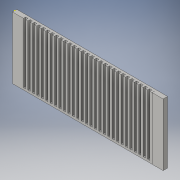
# Autodesk Inventor part: ModuleHolderReal
Saved by Autodesk Inventor 2016 (Build 200138000, 138)
## iProperties
Created: 2017-01-25
Part Number: ModuleHolderReal
Material: Generic
Document SubType Name: Modeling
Designer: RoboticsUser
Density: 1 g/cm^3
Appearance: Default
Author: RoboticsUser
Autodesk Inventor part; units mm, degrees
ref_plane "YZ Plane" through (0, 0, 0) normal (1, 0, 0) x (0, 1, 0)
ref_plane "XZ Plane" through (0, 0, 0) normal (0, 1, 0) x (-1, 0, 0)
ref_plane "XY Plane" through (0, 0, 0) normal (0, 0, 1) x (1, 0, 0)
sketch "Sketch1" plane through (0, 0, 0) normal (0, 0, 1) x (1, 0, 0)
  line L0 (0, 0) -> (215.9, 0)
  line L1 (215.9, 0) -> (215.9, -88.9)
  line L2 (215.9, -88.9) -> (0, -88.9)
  line L3 (0, -88.9) -> (0, 0)
  dimension "d0" = 215.9
  dimension "d1" = 88.9
  constraints: 8 end point, 2 parallel, 1 horizontal, 1 perpendicular
  measures "d0" distance of L1.end L2.end
  measures "d1" distance of L0.end L1.end
extrude "Extrusion1" add sketch "Sketch1" along normal blind 3.175
sketch "Sketch2" plane through (0, 0, 3.175) normal (0, 0, 1) x (1, 0, 0)
  line L0 (0, 0) -> (15.875, 0)
  line L1 (15.875, 0) -> (15.875, -88.9)
  line L2 (15.875, -88.9) -> (0, -88.9)
  line L3 (0, -88.9) -> (0, 0)
  dimension "d4" = 15.875
  dimension "d5" = 88.9
  constraints: 8 end point, 2 parallel, 1 horizontal, 1 perpendicular
  measures "d4" distance of L1.end L2.end
  measures "d5" distance of L0.end L1.end
extrude "Extrusion2" add sketch "Sketch2" along normal blind 3.175
sketch "Sketch3" plane through (0, 0, 3.175) normal (0, 0, 1) x (1, 0, 0)
  line L0 (215.9, -88.9) -> (0, -88.9) projected
  line L1 (15.8666, -88.9) -> (19.0416, -88.9)
  line L2 (19.0416, -88.9) -> (19.0416, -85.725)
  line L3 (19.0416, -85.725) -> (15.8666, -85.725)
  line L4 (15.8666, -85.725) -> (15.8666, -88.9)
  point P0 (0, 0)
  dimension "d8" = 3.175
  dimension "d9" = 3.175
  constraints: 8 end point, 2 parallel, 1 horizontal, 1 perpendicular, 1 point on line
  measures "d8" distance of L3.end L2.end
  measures "d9" distance of L2.end L1.end
extrude "Extrusion3" add sketch "Sketch3" along normal blind 3.175
sketch "Sketch4" plane through (0, 0, 3.175) normal (0, 0, 1) x (1, 0, 0)
  line L0 (19.0416, -85.725) -> (19.0416, -88.9) projected
  line L1 (19.0416, -88.9) -> (22.2166, -88.9)
  line L2 (22.2166, -88.9) -> (22.2166, 0)
  line L3 (22.2166, 0) -> (19.0416, 0)
  line L4 (19.0416, 0) -> (19.0416, -88.9)
  point P0 (0, 0)
  dimension "d12" = 3.175
  dimension "d13" = 88.9
  constraints: 8 end point, 2 parallel, 1 horizontal, 1 perpendicular
  measures "d12" distance of L3.end L2.end
  measures "d13" distance of L2.end L1.end
extrude "Extrusion4" add sketch "Sketch4" along normal blind 3.175
sketch "Sketch5" plane through (0, 0, 3.175) normal (0, 0, 1) x (1, 0, 0)
  line L0 (215.9, -88.9) -> (0, -88.9) projected
  line L1 (22.2165, -88.9) -> (25.3915, -88.9)
  line L2 (25.3915, -88.9) -> (25.3915, -85.725)
  line L3 (25.3915, -85.725) -> (22.2165, -85.725)
  line L4 (22.2165, -85.725) -> (22.2165, -88.9)
  point P0 (0, 0)
  dimension "d16" = 3.175
  dimension "d17" = 3.175
  constraints: 8 end point, 2 parallel, 1 horizontal, 1 perpendicular, 1 point on line
  measures "d16" distance of L3.end L2.end
  measures "d17" distance of L2.end L1.end
extrude "Extrusion5" add sketch "Sketch5" along normal blind 3.175
sketch "Sketch6" plane through (0, 0, 3.175) normal (0, 0, 1) x (1, 0, 0)
  point P0 (0, 0)
sketch "Sketch7" plane through (0, 0, 3.175) normal (0, 0, 1) x (1, 0, 0)
  line L0 (25.3915, -85.725) -> (25.3915, -88.9) projected
  line L1 (25.3915, -88.9) -> (28.5665, -88.9)
  line L2 (28.5665, -88.9) -> (28.5665, 0)
  line L3 (28.5665, 0) -> (25.3915, 0)
  line L4 (25.3915, 0) -> (25.3915, -88.9)
  point P0 (0, 0)
  dimension "d20" = 3.175
  dimension "d21" = 88.9
  constraints: 8 end point, 2 parallel, 1 horizontal, 1 perpendicular
  measures "d20" distance of L3.end L2.end
  measures "d21" distance of L2.end L1.end
extrude "Extrusion6" add sketch "Sketch7" along normal blind 3.175
sketch "Sketch8" plane through (0, 0, 3.175) normal (0, 0, 1) x (1, 0, 0)
  line L0 (28.5665, 0) -> (28.5665, -88.9) projected
  line L1 (28.5665, -88.9) -> (31.7415, -88.9)
  line L2 (31.7415, -88.9) -> (31.7415, -85.725)
  line L3 (31.7415, -85.725) -> (28.5665, -85.725)
  line L4 (28.5665, -85.725) -> (28.5665, -88.9)
  point P0 (0, 0)
  dimension "d24" = 3.175
  dimension "d25" = 3.175
  constraints: 8 end point, 2 parallel, 1 horizontal, 1 perpendicular
  measures "d24" distance of L3.end L2.end
  measures "d25" distance of L2.end L1.end
extrude "Extrusion7" add sketch "Sketch8" along normal blind 3.175
sketch "Sketch9" plane through (0, 0, 3.175) normal (0, 0, 1) x (1, 0, 0)
  line L0 (31.7415, -85.725) -> (31.7415, -88.9) projected
  line L1 (31.7415, -88.9) -> (34.9165, -88.9)
  line L2 (34.9165, -88.9) -> (34.9165, 0)
  line L3 (34.9165, 0) -> (31.7415, 0)
  line L4 (31.7415, 0) -> (31.7415, -88.9)
  point P0 (0, 0)
  dimension "d28" = 3.175
  dimension "d29" = 88.9
  constraints: 8 end point, 2 parallel, 1 horizontal, 1 perpendicular
  measures "d28" distance of L3.end L2.end
  measures "d29" distance of L2.end L1.end
extrude "Extrusion8" add sketch "Sketch9" along normal blind 3.175
sketch "Sketch10" plane through (0, 0, 3.175) normal (0, 0, 1) x (1, 0, 0)
  line L0 (215.9, -88.9) -> (215.9, 0) projected
  line L1 (215.9, -88.9) -> (200.025, -88.9)
  line L2 (200.025, -88.9) -> (200.025, 0)
  line L3 (200.025, 0) -> (215.9, 0)
  line L4 (215.9, 0) -> (215.9, -88.9)
  point P0 (0, 0)
  dimension "d32" = 15.875
  dimension "d33" = 88.9
  constraints: 8 end point, 2 parallel, 1 horizontal, 1 perpendicular
  measures "d32" distance of L2.end L3.end
  measures "d33" distance of L1.end L2.end
extrude "Extrusion9" add sketch "Sketch10" along normal blind 3.175
sketch "Sketch11" plane through (0, 0, 3.175) normal (0, 0, 1) x (1, 0, 0)
  line L0 (34.9165, 0) -> (34.9165, -88.9) projected
  line L1 (34.9165, -88.9) -> (38.0915, -88.9)
  line L2 (38.0915, -88.9) -> (38.0915, -85.725)
  line L3 (38.0915, -85.725) -> (34.9165, -85.725)
  line L4 (34.9165, -85.725) -> (34.9165, -88.9)
  point P0 (0, 0)
  dimension "d36" = 3.175
  dimension "d37" = 3.175
  constraints: 8 end point, 2 parallel, 1 horizontal, 1 perpendicular
  measures "d36" distance of L3.end L2.end
  measures "d37" distance of L2.end L1.end
extrude "Extrusion10" add sketch "Sketch11" along normal blind 3.175
sketch "Sketch12" plane through (0, 0, 3.175) normal (0, 0, 1) x (1, 0, 0)
  line L0 (38.0915, -88.9) -> (200.025, -88.9) projected
  line L1 (38.0915, -88.9) -> (41.2665, -88.9)
  line L2 (41.2665, -88.9) -> (41.2665, 0)
  line L3 (41.2665, 0) -> (38.0915, 0)
  line L4 (38.0915, 0) -> (38.0915, -88.9)
  point P0 (0, 0)
  dimension "d40" = 3.175
  dimension "d41" = 88.9
  constraints: 8 end point, 2 parallel, 1 horizontal, 1 perpendicular
  measures "d40" distance of L3.end L2.end
  measures "d41" distance of L2.end L1.end
extrude "Extrusion11" add sketch "Sketch12" along normal blind 3.175
sketch "Sketch13" plane through (0, 0, 3.175) normal (0, 0, 1) x (1, 0, 0)
  line L0 (41.2665, -88.9) -> (200.025, -88.9) projected
  line L1 (41.2665, -88.9) -> (44.4415, -88.9)
  line L2 (44.4415, -88.9) -> (44.4415, -85.725)
  line L3 (44.4415, -85.725) -> (41.2665, -85.725)
  line L4 (41.2665, -85.725) -> (41.2665, -88.9)
  point P0 (0, 0)
  dimension "d44" = 3.175
  dimension "d45" = 3.175
  constraints: 8 end point, 2 parallel, 1 horizontal, 1 perpendicular
  measures "d44" distance of L3.end L2.end
  measures "d45" distance of L2.end L1.end
extrude "Extrusion12" add sketch "Sketch13" along normal blind 3.175
sketch "Sketch14" plane through (0, 0, 3.175) normal (0, 0, 1) x (1, 0, 0)
  line L0 (44.4415, -88.9) -> (47.6165, -88.9)
  line L1 (47.6165, -88.9) -> (47.6165, 0)
  line L2 (47.6165, 0) -> (44.4415, 0)
  line L3 (44.4415, 0) -> (44.4415, -88.9)
  point P0 (0, 0)
  dimension "d48" = 3.175
  dimension "d49" = 88.9
  constraints: 8 end point, 2 parallel, 1 horizontal, 1 perpendicular
  measures "d48" distance of L2.end L1.end
  measures "d49" distance of L1.end L0.end
extrude "Extrusion13" add sketch "Sketch14" along normal blind 3.175
sketch "Sketch15" plane through (0, 0, 3.175) normal (0, 0, 1) x (1, 0, 0)
  line L0 (47.6165, -88.9) -> (200.025, -88.9) projected
  line L1 (47.6165, -88.9) -> (50.7915, -88.9)
  line L2 (50.7915, -88.9) -> (50.7915, -85.725)
  line L3 (50.7915, -85.725) -> (47.6165, -85.725)
  line L4 (47.6165, -85.725) -> (47.6165, -88.9)
  point P0 (0, 0)
  dimension "d52" = 3.175
  dimension "d53" = 3.175
  constraints: 8 end point, 2 parallel, 1 horizontal, 1 perpendicular
  measures "d52" distance of L3.end L2.end
  measures "d53" distance of L2.end L1.end
extrude "Extrusion14" add sketch "Sketch15" along normal blind 3.175
sketch "Sketch16" plane through (0, 0, 3.175) normal (0, 0, 1) x (1, 0, 0)
  line L0 (50.7915, -88.9) -> (200.025, -88.9) projected
  line L1 (50.7915, -88.9) -> (53.9665, -88.9)
  line L2 (53.9665, -88.9) -> (53.9665, 0)
  line L3 (53.9665, 0) -> (50.7915, 0)
  line L4 (50.7915, 0) -> (50.7915, -88.9)
  point P0 (0, 0)
  dimension "d56" = 3.175
  dimension "d57" = 88.9
  constraints: 8 end point, 2 parallel, 1 horizontal, 1 perpendicular
  measures "d56" distance of L3.end L2.end
  measures "d57" distance of L2.end L1.end
extrude "Extrusion15" add sketch "Sketch16" along normal blind 3.175
sketch "Sketch17" plane through (0, 0, 3.175) normal (0, 0, 1) x (1, 0, 0)
  line L0 (53.9665, -88.9) -> (200.025, -88.9) projected
  line L1 (53.9665, -88.9) -> (57.1415, -88.9)
  line L2 (57.1415, -88.9) -> (57.1415, -85.725)
  line L3 (57.1415, -85.725) -> (53.9665, -85.725)
  line L4 (53.9665, -85.725) -> (53.9665, -88.9)
  point P0 (0, 0)
  dimension "d60" = 3.175
  dimension "d61" = 3.175
  constraints: 8 end point, 2 parallel, 1 horizontal, 1 perpendicular
  measures "d60" distance of L3.end L2.end
  measures "d61" distance of L2.end L1.end
extrude "Extrusion16" add sketch "Sketch17" along normal blind 3.175
sketch "Sketch18" plane through (0, 0, 3.175) normal (0, 0, 1) x (1, 0, 0)
  line L0 (57.1415, -85.725) -> (57.1415, -88.9) projected
  line L1 (57.1415, -88.9) -> (60.3165, -88.9)
  line L2 (60.3165, -88.9) -> (60.3165, 0)
  line L3 (60.3165, 0) -> (57.1415, 0)
  line L4 (57.1415, 0) -> (57.1415, -88.9)
  point P0 (0, 0)
  dimension "d64" = 3.175
  dimension "d65" = 88.9
  constraints: 8 end point, 2 parallel, 1 horizontal, 1 perpendicular
  measures "d64" distance of L3.end L2.end
  measures "d65" distance of L2.end L1.end
extrude "Extrusion17" add sketch "Sketch18" along normal blind 3.175
sketch "Sketch19" plane through (0, 0, 3.175) normal (0, 0, 1) x (1, 0, 0)
  line L0 (60.3165, -88.9) -> (200.025, -88.9) projected
  line L1 (60.3165, -88.9) -> (63.4915, -88.9)
  line L2 (63.4915, -88.9) -> (63.4915, -85.725)
  line L3 (63.4915, -85.725) -> (60.3165, -85.725)
  line L4 (60.3165, -85.725) -> (60.3165, -88.9)
  point P0 (0, 0)
  dimension "d68" = 3.175
  dimension "d69" = 3.175
  constraints: 8 end point, 2 parallel, 1 horizontal, 1 perpendicular
  measures "d68" distance of L3.end L2.end
  measures "d69" distance of L2.end L1.end
extrude "Extrusion18" add sketch "Sketch19" along normal blind 3.175
sketch "Sketch20" plane through (0, 0, 3.175) normal (0, 0, 1) x (1, 0, 0)
  line L0 (63.4915, -85.725) -> (63.4915, -88.9) projected
  line L1 (63.4915, -88.9) -> (66.6665, -88.9)
  line L2 (66.6665, -88.9) -> (66.6665, 0)
  line L3 (66.6665, 0) -> (63.4915, 0)
  line L4 (63.4915, 0) -> (63.4915, -88.9)
  point P0 (0, 0)
  dimension "d72" = 3.175
  dimension "d73" = 88.9
  constraints: 8 end point, 2 parallel, 1 horizontal, 1 perpendicular
  measures "d72" distance of L3.end L2.end
  measures "d73" distance of L2.end L1.end
extrude "Extrusion19" add sketch "Sketch20" along normal blind 3.175
sketch "Sketch21" plane through (0, 0, 3.175) normal (0, 0, 1) x (1, 0, 0)
  line L0 (66.6665, -88.9) -> (200.025, -88.9) projected
  line L1 (66.6665, -88.9) -> (69.8415, -88.9)
  line L2 (69.8415, -88.9) -> (69.8415, -85.725)
  line L3 (69.8415, -85.725) -> (66.6665, -85.725)
  line L4 (66.6665, -85.725) -> (66.6665, -88.9)
  point P0 (0, 0)
  dimension "d76" = 3.175
  dimension "d77" = 3.175
  constraints: 8 end point, 2 parallel, 1 horizontal, 1 perpendicular
  measures "d76" distance of L3.end L2.end
  measures "d77" distance of L2.end L1.end
extrude "Extrusion20" add sketch "Sketch21" along normal blind 3.175
sketch "Sketch22" plane through (0, 0, 3.175) normal (0, 0, 1) x (1, 0, 0)
  line L0 (69.8415, -88.9) -> (200.025, -88.9) projected
  line L1 (69.8415, -88.9) -> (73.0165, -88.9)
  line L2 (73.0165, -88.9) -> (73.0165, 0)
  line L3 (73.0165, 0) -> (69.8415, 0)
  line L4 (69.8415, 0) -> (69.8415, -88.9)
  point P0 (0, 0)
  dimension "d80" = 3.175
  dimension "d81" = 88.9
  constraints: 8 end point, 2 parallel, 1 horizontal, 1 perpendicular
  measures "d80" distance of L3.end L2.end
  measures "d81" distance of L2.end L1.end
extrude "Extrusion21" add sketch "Sketch22" along normal blind 3.175
sketch "Sketch23" plane through (0, 0, 3.175) normal (0, 0, 1) x (1, 0, 0)
  line L0 (73.0165, -88.9) -> (200.025, -88.9) projected
  line L1 (73.0165, -88.9) -> (76.1915, -88.9)
  line L2 (76.1915, -88.9) -> (76.1915, -85.725)
  line L3 (76.1915, -85.725) -> (73.0165, -85.725)
  line L4 (73.0165, -85.725) -> (73.0165, -88.9)
  point P0 (0, 0)
  dimension "d84" = 3.175
  dimension "d85" = 3.175
  constraints: 8 end point, 2 parallel, 1 horizontal, 1 perpendicular
  measures "d84" distance of L3.end L2.end
  measures "d85" distance of L2.end L1.end
extrude "Extrusion22" add sketch "Sketch23" along normal blind 3.175
sketch "Sketch24" plane through (0, 0, 3.175) normal (0, 0, 1) x (1, 0, 0)
  line L0 (76.1915, -88.9) -> (200.025, -88.9) projected
  line L1 (76.1915, -88.9) -> (79.3665, -88.9)
  line L2 (79.3665, -88.9) -> (79.3665, 0)
  line L3 (79.3665, 0) -> (76.1915, 0)
  line L4 (76.1915, 0) -> (76.1915, -88.9)
  point P0 (0, 0)
  dimension "d88" = 3.175
  dimension "d89" = 88.9
  constraints: 8 end point, 2 parallel, 1 horizontal, 1 perpendicular
  measures "d88" distance of L3.end L2.end
  measures "d89" distance of L2.end L1.end
extrude "Extrusion23" add sketch "Sketch24" along normal blind 3.175
sketch "Sketch25" plane through (0, 0, 3.175) normal (0, 0, 1) x (1, 0, 0)
  line L0 (79.3665, -88.9) -> (82.5415, -88.9)
  line L1 (82.5415, -88.9) -> (82.5415, -85.725)
  line L2 (82.5415, -85.725) -> (79.3665, -85.725)
  line L3 (79.3665, -85.725) -> (79.3665, -88.9)
  point P0 (0, 0)
  dimension "d92" = 3.175
  dimension "d93" = 3.175
  constraints: 8 end point, 2 parallel, 1 horizontal, 1 perpendicular
  measures "d92" distance of L2.end L1.end
  measures "d93" distance of L1.end L0.end
extrude "Extrusion24" add sketch "Sketch25" along normal blind 3.175
sketch "Sketch26" plane through (0, 0, 3.175) normal (0, 0, 1) x (1, 0, 0)
  line L0 (82.5415, -85.725) -> (82.5415, -88.9) projected
  line L1 (82.5415, -88.9) -> (85.7165, -88.9)
  line L2 (85.7165, -88.9) -> (85.7165, 0)
  line L3 (85.7165, 0) -> (82.5415, 0)
  line L4 (82.5415, 0) -> (82.5415, -88.9)
  point P0 (0, 0)
  dimension "d96" = 3.175
  dimension "d97" = 88.9
  constraints: 8 end point, 2 parallel, 1 horizontal, 1 perpendicular
  measures "d96" distance of L3.end L2.end
  measures "d97" distance of L2.end L1.end
extrude "Extrusion25" add sketch "Sketch26" along normal blind 3.175
sketch "Sketch27" plane through (0, 0, 3.175) normal (0, 0, 1) x (1, 0, 0)
  line L0 (85.7165, -88.9) -> (200.025, -88.9) projected
  line L1 (85.7165, -88.9) -> (88.8915, -88.9)
  line L2 (88.8915, -88.9) -> (88.8915, -85.725)
  line L3 (88.8915, -85.725) -> (85.7165, -85.725)
  line L4 (85.7165, -85.725) -> (85.7165, -88.9)
  point P0 (0, 0)
  dimension "d100" = 3.175
  dimension "d101" = 3.175
  constraints: 8 end point, 2 parallel, 1 horizontal, 1 perpendicular
  measures "d100" distance of L3.end L2.end
  measures "d101" distance of L2.end L1.end
extrude "Extrusion26" add sketch "Sketch27" along normal blind 3.175
sketch "Sketch28" plane through (0, 0, 3.175) normal (0, 0, 1) x (1, 0, 0)
  line L0 (88.8915, -88.9) -> (200.025, -88.9) projected
  line L1 (88.8915, -88.9) -> (92.0665, -88.9)
  line L2 (92.0665, -88.9) -> (92.0665, 0)
  line L3 (92.0665, 0) -> (88.8915, 0)
  line L4 (88.8915, 0) -> (88.8915, -88.9)
  point P0 (0, 0)
  dimension "d104" = 3.175
  dimension "d105" = 88.9
  constraints: 8 end point, 2 parallel, 1 horizontal, 1 perpendicular
  measures "d104" distance of L3.end L2.end
  measures "d105" distance of L2.end L1.end
extrude "Extrusion27" add sketch "Sketch28" along normal blind 3.175
sketch "Sketch29" plane through (0, 0, 3.175) normal (0, 0, 1) x (1, 0, 0)
  line L0 (92.0665, -88.9) -> (200.025, -88.9) projected
  line L1 (92.0665, -88.9) -> (95.2415, -88.9)
  line L2 (95.2415, -88.9) -> (95.2415, -85.725)
  line L3 (95.2415, -85.725) -> (92.0665, -85.725)
  line L4 (92.0665, -85.725) -> (92.0665, -88.9)
  point P0 (0, 0)
  dimension "d108" = 3.175
  dimension "d109" = 3.175
  constraints: 8 end point, 2 parallel, 1 horizontal, 1 perpendicular
  measures "d108" distance of L3.end L2.end
  measures "d109" distance of L2.end L1.end
extrude "Extrusion28" add sketch "Sketch29" along normal blind 3.175
sketch "Sketch30" plane through (0, 0, 3.175) normal (0, 0, 1) x (1, 0, 0)
  line L0 (95.2415, -85.725) -> (95.2415, -88.9) projected
  line L1 (95.2415, -88.9) -> (98.4165, -88.9)
  line L2 (98.4165, -88.9) -> (98.4165, 0)
  line L3 (98.4165, 0) -> (95.2415, 0)
  line L4 (95.2415, 0) -> (95.2415, -88.9)
  point P0 (0, 0)
  dimension "d112" = 3.175
  dimension "d113" = 88.9
  constraints: 8 end point, 2 parallel, 1 horizontal, 1 perpendicular
  measures "d112" distance of L3.end L2.end
  measures "d113" distance of L2.end L1.end
extrude "Extrusion29" add sketch "Sketch30" along normal blind 3.175
sketch "Sketch31" plane through (0, 0, 3.175) normal (0, 0, 1) x (1, 0, 0)
  line L0 (98.4165, -88.9) -> (200.025, -88.9) projected
  line L1 (98.4165, -88.9) -> (101.5915, -88.9)
  line L2 (101.5915, -88.9) -> (101.5915, -85.7152)
  line L3 (101.5915, -85.7152) -> (98.4165, -85.7152)
  line L4 (98.4165, -85.7152) -> (98.4165, -88.9)
  point P0 (0, 0)
  dimension "d116" = 3.175
  constraints: 8 end point, 2 parallel, 1 horizontal, 1 perpendicular
  measures "d116" distance of L3.end L2.end
extrude "Extrusion30" add sketch "Sketch31" along normal blind 3.175
sketch "Sketch32" plane through (0, 0, 3.175) normal (0, 0, 1) x (1, 0, 0)
  line L0 (101.5915, -85.7152) -> (101.5915, -88.9) projected
  line L1 (101.5915, -88.9) -> (104.7665, -88.9)
  line L2 (104.7665, -88.9) -> (104.7665, 0)
  line L3 (104.7665, 0) -> (101.5915, 0)
  line L4 (101.5915, 0) -> (101.5915, -88.9)
  point P0 (0, 0)
  dimension "d119" = 3.175
  dimension "d120" = 88.9
  constraints: 8 end point, 2 parallel, 1 horizontal, 1 perpendicular
  measures "d119" distance of L3.end L2.end
  measures "d120" distance of L2.end L1.end
extrude "Extrusion31" add sketch "Sketch32" along normal blind 3.175
sketch "Sketch33" plane through (0, 0, 3.175) normal (0, 0, 1) x (1, 0, 0)
  line L0 (104.7665, -88.9) -> (200.025, -88.9) projected
  line L1 (104.7665, -88.9) -> (107.9415, -88.9)
  line L2 (107.9415, -88.9) -> (107.9415, -85.725)
  line L3 (107.9415, -85.725) -> (104.7665, -85.725)
  line L4 (104.7665, -85.725) -> (104.7665, -88.9)
  point P0 (0, 0)
  dimension "d123" = 3.175
  dimension "d124" = 3.175
  constraints: 8 end point, 2 parallel, 1 horizontal, 1 perpendicular
  measures "d123" distance of L3.end L2.end
  measures "d124" distance of L2.end L1.end
extrude "Extrusion32" add sketch "Sketch33" along normal blind 3.175
sketch "Sketch34" plane through (0, 0, 3.175) normal (0, 0, 1) x (1, 0, 0)
  line L0 (107.9415, -85.725) -> (107.9415, -88.9) projected
  line L1 (107.9415, -88.9) -> (111.1165, -88.9)
  line L2 (111.1165, -88.9) -> (111.1165, 0)
  line L3 (111.1165, 0) -> (107.9415, 0)
  line L4 (107.9415, 0) -> (107.9415, -88.9)
  point P0 (0, 0)
  dimension "d127" = 3.175
  dimension "d128" = 88.9
  constraints: 8 end point, 2 parallel, 1 horizontal, 1 perpendicular
  measures "d127" distance of L3.end L2.end
  measures "d128" distance of L2.end L1.end
extrude "Extrusion33" add sketch "Sketch34" along normal blind 3.175
sketch "Sketch35" plane through (0, 0, 3.175) normal (0, 0, 1) x (1, 0, 0)
  line L0 (111.1165, 0) -> (111.1165, -88.9) projected
  line L1 (111.1165, -88.9) -> (114.2915, -88.9)
  line L2 (114.2915, -88.9) -> (114.2915, -85.725)
  line L3 (114.2915, -85.725) -> (111.1165, -85.725)
  line L4 (111.1165, -85.725) -> (111.1165, -88.9)
  point P0 (0, 0)
  dimension "d131" = 3.175
  dimension "d132" = 3.175
  constraints: 8 end point, 2 parallel, 1 horizontal, 1 perpendicular
  measures "d131" distance of L3.end L2.end
  measures "d132" distance of L2.end L1.end
extrude "Extrusion34" add sketch "Sketch35" along normal blind 3.175
pattern_linear "Rectangular Pattern1" count 2 spacing 6.35 along (1, 0, 0) of "Extrusion33"
pattern_linear "Rectangular Pattern2" count 2 spacing 6.35 along (1, 0, 0) of "Extrusion34"
pattern_linear "Rectangular Pattern3" count 2 spacing 12.7 along (1, 0, 0) of "Extrusion33", "Rectangular Pattern1"
pattern_linear "Rectangular Pattern4" count 2 spacing 12.7 along (1, 0, 0) of "Extrusion34", "Rectangular Pattern2"
pattern_linear "Rectangular Pattern5" count 2 spacing 25.4 along (1, 0, 0) of "Extrusion33", "Rectangular Pattern1", "Rectangular Pattern3"
pattern_linear "Rectangular Pattern6" count 2 spacing 25.4 along (1, 0, 0) of "Extrusion34", "Rectangular Pattern2", "Rectangular Pattern4"
pattern_linear "Rectangular Pattern7" count 2 spacing 57.15 along (1, 0, 0) of "Extrusion31"
pattern_linear "Rectangular Pattern8" count 2 spacing 76.2 along (1, 0, 0) of "Extrusion27"
pattern_linear "Rectangular Pattern9" count 2 spacing 50.8 along (1, 0, 0) of "Extrusion34", "Rectangular Pattern2", "Rectangular Pattern4"
pattern_linear "Rectangular Pattern10" count 2 spacing 88.9 along (1, 0, 0) of "Extrusion30"
pattern_linear "Rectangular Pattern11" count 2 spacing 114.3 along (1, 0, 0) of "Extrusion24"
pattern_linear "Rectangular Pattern12" count 2 spacing 63.5 along (1, 0, 0) of "Extrusion33", "Rectangular Pattern1", "Rectangular Pattern3"
pattern_linear "Rectangular Pattern13" count 2 spacing 107.95 along (1, 0, 0) of "Extrusion27"
body "Solid1"
